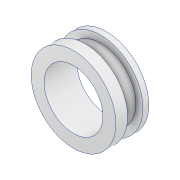
# Autodesk Inventor part: GT2_50teeth_25bore
Saved by Autodesk Inventor 2020 (Build 240168000, 168)
## iProperties
Created: 2019-05-05
Part Number: GT2_50teeth_25bore
Material: アルミニウム 6061
Document SubType Name: Modeling
Designer: ken113
Density: 2.7 g/cm^3
Appearance: アルミニウム - フラット
Mass: 14.4623 g
Surface Area: 42.3644 cm^2
Volume: 5.35642 cm^3
Author: ken113
Autodesk Inventor part; units mm, degrees
ref_plane "YZ Plane" through (0, 0, 0) normal (1, 0, 0) x (0, 1, 0)
ref_plane "XZ Plane" through (0, 0, 0) normal (0, 1, 0) x (-1, 0, 0)
sketch "スケッチ1" plane through (0, 0, 0) normal (0, 0, 1) x (1, 0, 0)
  circle A0 centre (0, 0) radius 12.5
  circle A1 centre (0, 0) radius 18
  dimension "d0" = 25
  dimension "d1" = 36
  constraints: 2 centre point, 2 coincident
  measures "d0" diameter of A0
  measures "d1" diameter of A1
extrude "押し出し1" add sketch "スケッチ1" along normal blind 14
ref_plane "作業平面1" through (0, 0, 9) normal (0, 0, 1) x (1, 0, 0)
sketch "スケッチ2" plane through (0, 0, 9) normal (0, 0, 1) x (1, 0, 0)
  circle A0 centre (0, 0) radius 15
  circle A1 centre (0, 0) radius 18
  dimension "d5" = 30
  constraints: 2 centre point, 2 coincident
  measures "d5" diameter of A0
extrude "押し出し2" cut sketch "スケッチ2" against normal blind 6.5
